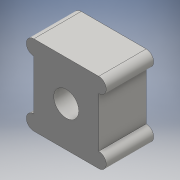
# Autodesk Inventor part: Varia
Saved by Autodesk Inventor 2016 (Build 200138000, 138)
## iProperties
Created: 2016-12-04
Part Number: Varia
Material: Generic
Document SubType Name: Modeling
Designer: Muhammad
Density: 1 g/cm^3
Appearance: Default
Author: Muhammad
Autodesk Inventor part; units mm, degrees
ref_plane "YZ Plane" through (0, 0, 0) normal (1, 0, 0) x (0, 1, 0)
ref_plane "XZ Plane" through (0, 0, 0) normal (0, 1, 0) x (-1, 0, 0)
ref_plane "XY Plane" through (0, 0, 0) normal (0, 0, 1) x (1, 0, 0)
sketch "Sketch1" plane through (0, 0, 0) normal (0, 1, 0) x (-1, 0, 0)
  line L0 (6.5, 8) -> (-6.5, 8)
  line L1 (-6.5, 5) -> (-6.5, -5)
  line L2 (-6.5, -8) -> (6.5, -8)
  line L3 (6.5, -5) -> (6.5, 5)
  line L4 (6.5, 8) -> (-6.5, -8) construction
  line L5 (-6.5, 8) -> (6.5, -8) construction
  arc A0 (6.5, 5) -> (6.5, 8) centre (6.5, 6.5) ccw
  arc A1 (6.5, -8) -> (6.5, -5) centre (6.5, -6.5) ccw
  arc A2 (-6.5, -5) -> (-6.5, -8) centre (-6.5, -6.5) ccw
  arc A3 (-6.5, 8) -> (-6.5, 5) centre (-6.5, 6.5) ccw
  point P0 (0, 0)
  dimension "d1" = 16
  constraints: 12 end point, 8 point on circle, 4 centre point, 2 midpoint, 2 parallel, 2 point on line, 1 horizontal, 1 perpendicular
  measures "d1" distance of L0.end L2.start
extrude "Extrusion1" add sketch "Sketch1" along normal mid plane 9.5
sketch "Sketch2" plane through (0, 4.75, 0) normal (0, 1, 0) x (1, 0, 0)
  circle A0 centre (0, 0) radius 2.5
  dimension "d6" = 5
  constraints: 1 centre point, 1 coincident
  measures "d6" diameter of A0
extrude "Extrusion2" cut sketch "Sketch2" against normal through all
body "Solid1"
